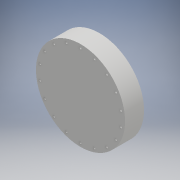
# Autodesk Inventor part: Korbbogenboden
Saved by Autodesk Inventor 2017 (Build 210142000, 142)
## iProperties
Created: 2019-06-21
Part Number: Korbbogenboden
Material: Generic
Document SubType Name: Modeling
Designer: Ole Simmering
Density: 1 g/cm^3
Appearance: Default
Author: Ole Simmering
Autodesk Inventor part; units mm, degrees
ref_plane "YZ Plane" through (0, 0, 0) normal (1, 0, 0) x (0, 1, 0)
ref_plane "XZ Plane" through (0, 0, 0) normal (0, 1, 0) x (-1, 0, 0)
ref_plane "XY Plane" through (0, 0, 0) normal (0, 0, 1) x (1, 0, 0)
sketch "Sketch1" plane through (0, 0, 0) normal (0, 0, 1) x (1, 0, 0)
  line L0 (0, -151.6511) -> (0, 29.6511) construction
  line L1 (144, 0) -> (144, -25)
  arc A0 (123.5827, -49.5764) -> (144, -25) centre (119, -25) ccw
  arc A1 (0, -61) -> (123.5827, -49.5764) centre (0, 613.1818) ccw
  line L2 (144, 0) -> (190, 0)
  line L3 (144, -25) -> (119, -25) construction
  line L4 (123.5827, -49.5764) -> (119, -25) construction
  line L5 (0, -61) -> (0, -81)
  line L6 (0, -81) -> (190, -81)
  line L7 (190, -81) -> (190, 0)
  point P0 (0, 0)
  dimension "d0" = 288
  dimension "d3" = 25
  dimension "d5" = 25
  dimension "d19" = 380
  dimension "d20" = 20
  dimension "d21" = 61
  constraints: 16 end point, 4 point on circle, 3 horizontal, 3 point on line, 2 centre point, 2 tangent, 2 vertical, 1 collinear, 1 line through centre, 1 midpoint, 1 perpendicular
  measures "d0" diameter of L1 L0
  measures "d3" radius of A0
  measures "d5" distance of L1.start L1.end
  measures "d19" diameter of L7 L0
  measures "d20" distance of L5.start L5.end
  measures "d21" distance of L5.start point (0, 0)
revolve "Revolution1" add sketch "Sketch1" angle 360 about axis through (0, -151.6511, 0) along (0, 1, 0)
sketch "Sketch2" plane through (0, 0, 0) normal (0, 1, 0) x (1, 0, 0)
  point P0 (0, 0)
  point P1 (0, -175)
  point P2 (0, 0)
  dimension "d8" = 175
  constraints: 1 coincident
  measures "d8" distance of point (0, 0) point (0, -175)
hole "Hole1" at (0, 0, 175) direction (0, -1, 0) diameter 8.376 end through all thread size "M10x1.5" class "6H" standard "ISO Metric profile"
pattern_circular "Circular Pattern1" count 18 over 360 about axis through (0, -12.5, 0) along (0, 1, 0) of "Hole1"
body "Solid1"
